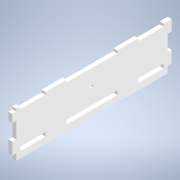
# Autodesk Inventor part: case top sides
Saved by Autodesk Inventor 2022 (Build 260153000, 153)
## iProperties
Created: 2021-05-28
Part Number: case top sides
Material: ABS Plastic
Document SubType Name: Modeling
Designer: benka
Density: 1.06 g/cm^3
Appearance: Smooth - White
Author: benka
Autodesk Inventor part; units mm, degrees
ref_plane "YZ Plane" through (0, 0, 0) normal (1, 0, 0) x (0, 1, 0)
ref_plane "XZ Plane" through (0, 0, 0) normal (0, 1, 0) x (-1, 0, 0)
ref_plane "XY Plane" through (0, 0, 0) normal (0, 0, 1) x (1, 0, 0)
sketch "Sketch1" plane through (0, 0, 0) normal (1, 0, 0) x (0, 1, 0)
  ellipse E0 centre (0, 0) end of major axis (0, -2) minor radius 1.9928
  line L0 (-20.007, -58.0002) -> (-20.007, -89.2502) projected
  line L1 (-20.007, -89.2502) -> (-25.007, -89.2502) projected
  line L2 (-25.007, -58.0002) -> (-25.007, -89.2502) projected
  line L3 (-20.007, -58.0002) -> (-25.007, -58.0002) projected
  line L4 (-20.007, 31.2498) -> (-20.007, -31.7502) projected
  line L5 (-20.007, -31.7502) -> (-25.007, -31.7502) projected
  line L6 (-25.007, 31.2498) -> (-25.007, -31.7502) projected
  line L7 (-20.007, 31.2498) -> (-25.007, 31.2498) projected
  line L8 (-20.007, 88.7498) -> (-20.007, 57.4998) projected
  line L9 (-20.007, 57.4998) -> (-25.007, 57.4998) projected
  line L10 (-25.007, 88.7498) -> (-25.007, 57.4998) projected
  line L11 (-20.007, 88.7498) -> (-25.007, 88.7498) projected
  line L12 (-25.0077, 93.7498) -> (-25.0077, 98.7498) projected
  line L13 (-10.0085, 98.7498) -> (-25.0077, 98.7498) projected
  line L14 (-10.0085, 93.7498) -> (-10.0085, 98.7498) projected
  line L15 (9.9915, 93.7498) -> (9.9915, 98.7498) projected
  line L16 (19.993, 98.7498) -> (9.9915, 98.7498) projected
  line L17 (9.9915, 93.7498) -> (-10.0085, 93.7498)
  line L18 (-25.0077, 93.7498) -> (-33.0079, 93.7498)
  line L19 (22.993, -99.2777) -> (9.993, -99.2502)
  line L20 (9.993, -99.2502) -> (9.993, -94.2502) projected
  line L21 (9.993, -94.2502) -> (-10.0077, -94.2502) projected
  line L22 (-10.0077, -99.2502) -> (-10.0077, -94.2502) projected
  line L23 (-10.0077, -99.2502) -> (-25.0077, -99.2502) projected
  line L24 (-25.0077, -99.2502) -> (-25.0077, -94.2502) projected
  line L25 (-25.0077, -94.2502) -> (-33.0079, -94.2502) projected
  line L26 (-33.0079, -94.2502) -> (-33.0079, 93.7498)
  line L27 (22.993, -99.2777) -> (22.993, -94.2502)
  line L28 (22.993, -89.2502) -> (22.993, -94.2502)
  line L29 (22.993, -89.2502) -> (19.993, -89.2502)
  line L30 (19.993, -58.0002) -> (19.993, -89.2502)
  line L31 (22.993, -58.0002) -> (19.993, -58.0002)
  line L32 (22.993, -31.7502) -> (22.993, -58.0002)
  line L33 (22.993, -31.7502) -> (19.993, -31.7502)
  line L34 (19.993, 31.2498) -> (19.993, -31.7502)
  line L35 (22.993, 31.2498) -> (19.993, 31.2498)
  line L36 (22.993, 57.4998) -> (22.993, 31.2498)
  line L37 (22.993, 57.4998) -> (19.993, 57.4998)
  line L38 (19.993, 88.7498) -> (19.993, 57.4998)
  line L39 (22.993, 88.7498) -> (19.993, 88.7498)
  line L40 (22.993, 93.7498) -> (22.993, 88.7498)
  line L41 (22.993, 93.7498) -> (19.993, 93.7498)
  line L42 (19.993, 93.7498) -> (19.993, 98.7498)
  point P0 (-29.9123, 87.1698)
  dimension "d21" = 188
  dimension "d26" = 3
  constraints: 40 end point, 7 collinear, 1 horizontal, 1 vertical, 3 other
  measures "d21" distance of L25.end L18.end
  measures "d26" distance between parallel lines of L32 L30
extrude "Extrusion1" add sketch "Sketch1" along normal blind 5
body "Solid1"
